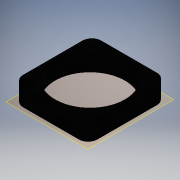
# Autodesk Inventor part: 02_Coolingfan
Saved by Autodesk Inventor 2016 (Build 200138000, 138)
## iProperties
Created: 2016-11-08
Part Number: 02_Coolingfan
Material: Generisch
Document SubType Name: Modeling
Designer: Bene
Density: 1 g/cm^3
Appearance: Schwarz
Author: Bene
Autodesk Inventor part; units mm, degrees
ref_plane "YZ Plane" through (0, 0, 0) normal (1, 0, 0) x (0, 1, 0)
ref_plane "XZ Plane" through (0, 0, 0) normal (0, 1, 0) x (-1, 0, 0)
ref_plane "XY Plane" through (0, 0, 0) normal (0, 0, 1) x (1, 0, 0)
ref_plane "Arbeitsebene1" through (0, 0, 0) normal (0, 0, 1) x (1, 0, 0)
sketch "Skizze1" plane through (0, 0, 0) normal (0, 0, 1) x (1, 0, 0)
  line L0 (0, 0) -> (40, 0) projected
  line L1 (40, 0) -> (40, 42) projected
  line L2 (0, 42) -> (40, 42) projected
  line L3 (0, 0) -> (0, 42) projected
  line L4 (5, 42) -> (35, 42)
  line L5 (40, 37) -> (40, 5)
  line L6 (35, 0) -> (5, 0)
  line L7 (0, 5) -> (0, 37)
  line L8 (0, 42) -> (40, 0) construction
  line L9 (40, 42) -> (0, 0) construction
  arc A0 (5, 42) -> (0, 37) centre (5, 37) ccw
  arc A1 (40, 37) -> (35, 42) centre (35, 37) ccw
  arc A2 (35, 0) -> (40, 5) centre (35, 5) ccw
  arc A3 (0, 5) -> (5, 0) centre (5, 5) ccw
  point P0 (20, 21)
  dimension "d0" = 5
  constraints: 12 end point, 8 point on circle, 8 point on line, 8 tangent, 4 centre point, 3 equal radius, 2 midpoint, 2 parallel, 1 horizontal, 1 perpendicular
  measures "d0" radius of A0
extrude "Extrusion1" add sketch "Skizze1" along normal blind 10 contours A3 L3 A0 L2 A1 L1 A2 L0
sketch "Skizze2" plane through (0, 0, 10) normal (0, 0, 1) x (1, 0, 0)
  line L0 (0, 37) -> (0, 5) projected
  arc A0 (0, 5) -> (5, 0) centre (5, 5) ccw projected
  line L1 (5, 0) -> (35, 0) projected
  arc A1 (35, 0) -> (40, 5) centre (35, 5) ccw projected
  line L2 (40, 5) -> (40, 37) projected
  arc A2 (40, 37) -> (35, 42) centre (35, 37) ccw projected
  line L3 (35, 42) -> (5, 42) projected
  arc A3 (5, 42) -> (0, 37) centre (5, 37) ccw projected
  circle A4 centre (20, 21) radius 18.75
  point P0 (0, 0)
  dimension "d3" = 37.5
  constraints: 1 centre point
  measures "d3" diameter of A4
extrude "Extrusion2" cut sketch "Skizze2" against normal through all contours A4
sketch "Skizze3" plane through (0, 0, 10) normal (0, 0, 1) x (1, 0, 0)
  circle A0 centre (20, 21) radius 18.75 projected
  line L0 (0, 37) -> (0, 5) projected
  arc A1 (0, 5) -> (5, 0) centre (5, 5) ccw projected
  line L1 (5, 0) -> (35, 0) projected
  arc A2 (35, 0) -> (40, 5) centre (35, 5) ccw projected
  line L2 (40, 5) -> (40, 37) projected
  arc A3 (40, 37) -> (35, 42) centre (35, 37) ccw projected
  line L3 (35, 42) -> (5, 42) projected
  arc A4 (5, 42) -> (0, 37) centre (5, 37) ccw projected
  circle A5 centre (5, 37) radius 1
  circle A6 centre (35, 37) radius 1
  circle A7 centre (35, 5) radius 1
  circle A8 centre (5, 5) radius 1
  point P0 (0, 0)
  dimension "d6" = 2
  dimension "d7" = 2
  dimension "d8" = 2
  dimension "d9" = 2
  constraints: 4 centre point, 4 coincident
  measures "d6" diameter of A5
  measures "d7" diameter of A6
  measures "d8" diameter of A7
  measures "d9" diameter of A8
extrude "Extrusion3" cut sketch "Skizze3" against normal through all contours A5 | A6 | A7 | A8
